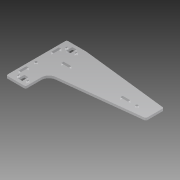
# Autodesk Inventor part: plastic_part_51
Saved by Autodesk Inventor 2013 (Build 170138000, 138)
## iProperties
Shininess: 20.0
Created: 2013-06-30
Part Number: plastic_part_51
Document SubType Name: Modeling
Designer: Noa Izumi
Material: Default
Density: 1 g/cm^3
Density: 0.0
Volumn: 0.0
Area: 0.0
PropertySet Name: Model Information
Control State: 0
Master: False
Checked Out: False
Author: Noa Izumi
Autodesk Inventor part; units mm, degrees
ref_plane "YZ Plane" through (0, 0, 0) normal (1, 0, 0) x (0, 1, 0)
ref_plane "XZ Plane" through (0, 0, 0) normal (0, 1, 0) x (-1, 0, 0)
ref_plane "XY Plane" through (0, 0, 0) normal (0, 0, 1) x (1, 0, 0)
sketch "Sketch1" plane through (0, 0, 0) normal (0, 0, 1) x (1, 0, 0)
  line L0 (0, 0) -> (25, 0)
  line L1 (25, 78) -> (0, 78)
  line L2 (0, 78) -> (0, 0)
  line L3 (11.354, 12) -> (16.646, 12)
  line L4 (16.646, 12) -> (16.646, 4)
  line L5 (16.646, 4) -> (11.354, 4)
  line L6 (11.354, 4) -> (11.354, 12)
  line L7 (11.354, 74) -> (16.646, 74)
  line L8 (16.646, 74) -> (16.646, 66)
  line L9 (16.646, 66) -> (11.354, 66)
  line L10 (11.354, 66) -> (11.354, 74)
  line L11 (138, 65) -> (138, 42)
  line L12 (25, 29) -> (138, 42)
  line L13 (25, 78) -> (138, 65)
  line L14 (25, 78) -> (25, 29)
  line L15 (25, 78) -> (25, 0)
  dimension "d0" = 25
  dimension "d1" = 78
  dimension "d2" = 4
  dimension "d3" = 4
  dimension "d4" = 8
  dimension "d5" = 8
  dimension "d6" = 5.292
  dimension "d8" = 5.292
  dimension "d12" = 23
  dimension "d84" = 13
  dimension "d91" = 13
  dimension "d123" = 113
  dimension "d146" = 8.354
  dimension "d147" = 25
  dimension "d148" = 8.354
  constraints: 32 end point, 6 parallel, 3 horizontal, 2 perpendicular, 1 collinear
  measures "d0" distance of L0.start L0.end
  measures "d1" distance of L1.end L0.start
  measures "d2" distance between parallel lines of L7 L1
  measures "d3" distance between parallel lines of L0 L5
  measures "d4" distance of L5.end L3.start
  measures "d5" distance of L9.end L7.start
  measures "d6" distance of L7.start L7.end
  measures "d8" distance of L3.start L3.end
  measures "d12" distance of L11.end L11.start
  measures "d84" vertical distance of L11.end L12.start
  measures "d91" vertical distance of L1.start L11.start
  measures "d123" distance between parallel lines of L11 L15
  measures "d146" distance between parallel lines of L15 L4
  measures "d147" distance of L1.start L1.end
  measures "d148" distance between parallel lines of L15 L8
extrude "Extrusion1" add sketch "Sketch1" along normal blind 3
fillet "Fillet1" radius 2 5 edges at (0, 0, 1.5) (0, 78, 1.5) (138, 65, 1.5) (138, 42, 1.5) (25, 0, 1.5)
fillet "Fillet3" radius 10 2 edges at (25, 29, 1.5) (25, 78, 1.5)
sketch "Sketch8" plane through (0, 0, 3) normal (0, 0, 1) x (1, 0, 0)
  line L0 (16.646, 12) -> (16.646, 4) projected
  line L1 (11.354, 4) -> (11.354, 12) projected
  line L2 (7.3, 68.75) -> (8.7, 68.75)
  line L3 (8.7, 68.75) -> (8.7, 71.25)
  line L4 (8.7, 71.25) -> (7.3, 71.25)
  line L5 (7.3, 71.25) -> (7.3, 68.75)
  line L6 (19.3, 71.25) -> (20.7, 71.25)
  line L7 (20.7, 71.25) -> (20.7, 68.75)
  line L8 (20.7, 68.75) -> (19.3, 68.75)
  line L9 (19.3, 68.75) -> (19.3, 71.25)
  line L10 (7.3, 6.75) -> (8.7, 6.75)
  line L11 (8.7, 6.75) -> (8.7, 9.25)
  line L12 (8.7, 9.25) -> (7.3, 9.25)
  line L13 (7.3, 9.25) -> (7.3, 6.75)
  line L14 (20.7, 6.75) -> (19.3, 6.75)
  line L15 (19.3, 6.75) -> (19.3, 9.25)
  line L16 (19.3, 9.25) -> (20.7, 9.25)
  line L17 (20.7, 9.25) -> (20.7, 6.75)
  line L18 (16.646, 74) -> (16.646, 66) projected
  line L19 (11.354, 66) -> (11.354, 74) projected
  line L20 (11.354, 74) -> (16.646, 74) projected
  line L21 (11.354, 12) -> (16.646, 12) projected
  dimension "d98" = 2.5
  dimension "d104" = 2.5
  dimension "d105" = 2.654
  dimension "d106" = 1.4
  dimension "d108" = 1.4
  dimension "d109" = 2.654
  dimension "d175" = 2.654
  dimension "d176" = 2.654
  dimension "d177" = 1.4
  dimension "d178" = 1.4
  dimension "d179" = 2.5
  dimension "d180" = 2.75
  dimension "d181" = 2.75
  dimension "d182" = 2.5
  dimension "d183" = 2.75
  dimension "d184" = 2.75
  constraints: 32 end point, 8 parallel, 4 horizontal, 4 perpendicular
  measures "d98" distance of L4.end L2.start
  measures "d104" distance of L12.end L10.start
  measures "d105" distance between parallel lines of L0 L15
  measures "d106" distance of L14.start L14.end
  measures "d108" distance of L10.start L10.end
  measures "d109" distance between parallel lines of L1 L11
  measures "d175" distance between parallel lines of L19 L3
  measures "d176" distance between parallel lines of L9 L18
  measures "d177" distance of L2.start L2.end
  measures "d178" distance of L7.end L8.end
  measures "d179" distance of L6.end L7.end
  measures "d180" distance between parallel lines of L4 L20
  measures "d181" distance between parallel lines of L6 L20
  measures "d182" distance of L16.end L14.start
  measures "d183" distance between parallel lines of L12 L21
  measures "d184" distance between parallel lines of L16 L21
extrude "Extrusion5" cut sketch "Sketch8" against normal through all
sketch "草圖13" plane through (0, 0, 3) normal (0, 0, 1) x (1, 0, 0)
  line L0 (2, 78) -> (24.4267, 78) projected
  line L1 (0, 2) -> (0, 76) projected
  line L2 (23, 0) -> (2, 0) projected
  line L3 (138, 63.2169) -> (138, 43.7831) projected
  line L4 (3, 65) -> (6, 65)
  line L5 (6, 65) -> (6, 55)
  line L6 (6, 55) -> (3, 55)
  line L7 (3, 55) -> (3, 65)
  line L8 (3, 23) -> (6, 23)
  line L9 (6, 23) -> (6, 13)
  line L10 (6, 13) -> (3, 13)
  line L11 (3, 13) -> (3, 23)
  line L12 (22, 52) -> (32, 52)
  line L13 (32, 52) -> (32, 49)
  line L14 (32, 49) -> (22, 49)
  line L15 (22, 49) -> (22, 52)
  line L16 (98, 52) -> (108, 52)
  line L17 (108, 52) -> (108, 49)
  line L18 (108, 49) -> (98, 49)
  line L19 (98, 49) -> (98, 52)
  point P0 (0, 0)
  dimension "d150" = 13
  dimension "d151" = 10
  dimension "d152" = 3
  dimension "d153" = 3
  dimension "d154" = 3
  dimension "d155" = 10
  dimension "d156" = 13
  dimension "d157" = 26
  dimension "d158" = 3
  dimension "d159" = 10
  dimension "d160" = 22
  dimension "d161" = 3
  dimension "d162" = 10
  dimension "d163" = 30
  constraints: 32 end point, 8 parallel, 4 horizontal, 4 perpendicular
  measures "d150" distance between parallel lines of L0 L4
  measures "d151" distance of L6.end L4.start
  measures "d152" distance of L5.end L6.end
  measures "d153" distance between parallel lines of L7 L1
  measures "d154" distance of L8.start L8.end
  measures "d155" distance of L10.end L8.start
  measures "d156" distance between parallel lines of L2 L10
  measures "d157" distance between parallel lines of L12 L0
  measures "d158" distance of L14.end L12.start
  measures "d159" distance of L13.end L14.end
  measures "d160" distance between parallel lines of L1 L15
  measures "d161" distance of L18.end L16.start
  measures "d162" distance of L17.end L18.end
  measures "d163" distance between parallel lines of L3 L17
extrude "擠出7" cut sketch "草圖13" against normal through all
sketch "草圖14" plane through (0, 0, 3) normal (0, 0, 1) x (1, 0, 0)
  line L0 (23, 0) -> (2, 0) projected
  line L1 (138, 63.2169) -> (138, 43.7831) projected
  point P0 (0, 0)
  point P1 (118, 50.5)
  point P2 (4.5, 34)
  dimension "d166" = 20
  dimension "d167" = 34
  measures "d166" distance from line of L1 point (118, 50.5)
  measures "d167" distance from line of L0 point (4.5, 34)
hole "孔4" at (118, 50.5, 3) at (4.5, 34, 3) direction (0, 0, -1) diameter 3 end through all
